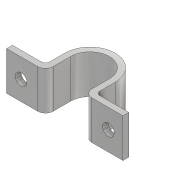
# Autodesk Inventor part: Part2
Saved by Autodesk Inventor 2017 (Build 210142000, 142)
## iProperties
Created: 2023-11-15
Part Number: Part2
Material: Generic
Document SubType Name: Modeling
Designer: Ok
Density: 1 g/cm^3
Appearance: Aluminum - Polished
Author: Ok
Autodesk Inventor part; units mm, degrees
ref_plane "YZ Plane" through (0, 0, 0) normal (1, 0, 0) x (0, 1, 0)
ref_plane "XZ Plane" through (0, 0, 0) normal (0, 1, 0) x (-1, 0, 0)
ref_plane "XY Plane" through (0, 0, 0) normal (0, 0, 1) x (1, 0, 0)
sketch "Sketch1" plane through (0, 0, 0) normal (0, 0, 1) x (1, 0, 0)
  arc A0 (5, 0) -> (0, 5) centre (0, 0) ccw
  arc A1 (6.5, 0) -> (0, 6.5) centre (0, 0) ccw
  line L0 (7, -6.5) -> (15, -6.5)
  line L1 (7.5, -5) -> (15, -5)
  line L2 (15, -5) -> (15, -6.5)
  line L3 (6.5, 0) -> (6.5, -4)
  line L4 (5, 0) -> (5, -4.5)
  arc A2 (5, -4.5) -> (7, -6.5) centre (7, -4.5) ccw
  arc A3 (6.5, -4) -> (7.5, -5) centre (7.5, -4) ccw
  arc A4 (0, 5) -> (-5, 0) centre (0, 0) ccw
  arc A5 (0, 6.5) -> (-6.5, 0) centre (0, 0) ccw
  line L5 (-7, -6.5) -> (-15, -6.5)
  line L6 (-7.5, -5) -> (-15, -5)
  line L7 (-15, -5) -> (-15, -6.5)
  line L8 (-6.5, 0) -> (-6.5, -4)
  line L9 (-5, 0) -> (-5, -4.5)
  arc A6 (-7, -6.5) -> (-5, -4.5) centre (-7, -4.5) ccw
  arc A7 (-7.5, -5) -> (-6.5, -4) centre (-7.5, -4) ccw
  point P0 (0, -12.0627)
  dimension "d0" = 10
  dimension "d1" = 1.5
  dimension "d2" = 2
  dimension "d3" = 1
  constraints: 20 end point, 16 point on circle, 8 centre point, 4 tangent, 2 coincident, 2 horizontal, 2 perpendicular, 1 vertical
  measures "d0" diameter of A0
  measures "d1" radial gap between concentric circles of A0 A1
  measures "d2" radius of A2
  measures "d3" radius of A3
extrude "Extrusion1" add sketch "Sketch1" along normal mid plane 10
sketch "Sketch2" plane through (7.5, -5, 5) normal (0, 1, 0) x (1, 0, 0)
  circle A0 centre (-18.75, 5) radius 1.5
  line L0 (-22.5, 0) -> (-22.5, 10) projected
  line L1 (-7.5, -2.4485) -> (-7.5, 17.5561) construction
  circle A1 centre (3.75, 5) radius 1.5
  point P0 (-7.5, 5)
  dimension "d6" = 3
  dimension "d7" = 3.75
  constraints: 2 centre point, 2 end point, 1 symmetric about line, 1 vertical, 1 other
  measures "d6" diameter of A0
  measures "d7" distance from line of L0 A0.centre
extrude "Extrusion2" cut sketch "Sketch2" against normal up to next
body "Solid1"
